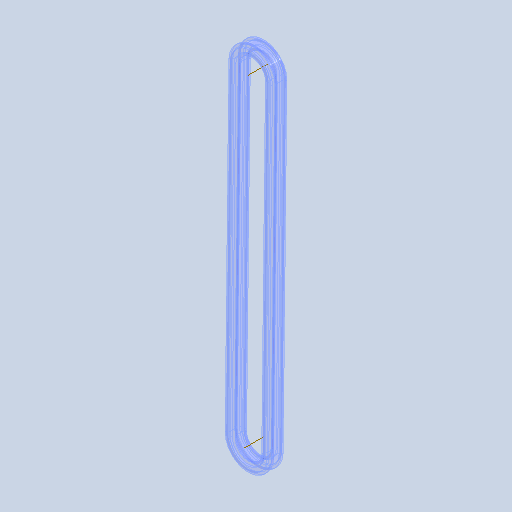
# Autodesk Inventor part: Cadena de rodillos
Saved by Autodesk Inventor 2022.1 (Build 261234000, 234)
## iProperties
Created: 2021-09-11
Part Number: Cadena de rodillos
Material: Generic
Document SubType Name: Modeling
Designer: seb_0
Density: 1 g/cm^3
Appearance: Clear - Blue
CustomPartVersion: 1
Author: seb_0
Autodesk Inventor part; units mm, degrees
ref_plane "Plano de trabajo2" through (36.0243, 99.5749, 0) normal (-1, 0, 0) x (0, 0, 1)
ref_plane "Plano de trabajo3" through (27.084, -687.8643, 0) normal (0.415415, 0.909632, 0) x (0, 0, 1)
sketch "Trayectoria" plane through (0, 0, 0) normal (0, 0, 1) x (1, 0, 0)
  arc A0 (80.3897, 99.0711) -> (-8.3412, 100.0786) centre (36.0243, 99.5749) ccw
  arc A1 (-17.2814, -687.3606) -> (71.4495, -688.3681) centre (27.084, -687.8643) ccw
  line L0 (-17.2814, -687.3606) -> (-8.3412, 100.0786)
  line L1 (80.3897, 99.0711) -> (71.4495, -688.3681)
  dimension "d31" = 24
  constraints: 4 end point, 4 point on circle, 2 centre point
ref_plane "Plano de sección" through (-8.3412, 100.0786, 0) normal (-0.0113528, -0.9999356, 0) x (0, 0, 1)
sketch "Boceto de sección" plane through (-8.3412, 100.0786, 0) normal (-0.0113528, -0.9999356, 0) x (0, 0, 1)
  line L0 (-18, -5) -> (18, -5)
  line L1 (18, -5) -> (18, 5)
  line L2 (18, 5) -> (-18, 5)
  line L3 (-18, 5) -> (-18, -5)
  line L4 (-9, -7.5) -> (9, -7.5)
  line L5 (9, -7.5) -> (9, 7.5)
  line L6 (9, 7.5) -> (-9, 7.5)
  line L7 (-9, 7.5) -> (-9, -7.5)
  line L8 (-9, 0) -> (9, 0) construction
  line L9 (-14, -12) -> (-9, -12)
  line L10 (-9, -12) -> (-9, 12)
  line L11 (-9, 12) -> (-14, 12)
  line L12 (-14, 12) -> (-14, -12)
  line L13 (9, -12) -> (14, -12)
  line L14 (14, -12) -> (14, 12)
  line L15 (14, 12) -> (9, 12)
  line L16 (9, 12) -> (9, -12)
  line L17 (-18, 0) -> (18, 0) construction
  point P0 (0, 0)
  point P1 (0, 0)
  dimension "d21" = 10
  dimension "d22" = 15
  dimension "d23" = 18
  dimension "d24" = 5
  dimension "d31" = 24
  dimension "d32" = 36
  constraints: 36 end point, 8 midpoint, 8 parallel, 4 horizontal, 4 perpendicular, 3 collinear, 1 coincident, 1 other
  measures "d21" distance between parallel lines of L2 L0
  measures "d22" distance between parallel lines of L6 L4
  measures "d23" distance between parallel lines of L5 L7
  measures "d24" distance between parallel lines of L12 L10
  measures "d31" distance between parallel lines of L11 L9
  measures "d32" distance between parallel lines of L1 L3
sweep "Sólido" add profiles "Boceto de sección" path "Trayectoria" path curves L1 A1 L0 A0
pattern_of_one "Strand Pattern"
equation "\"d21\" = da_d2"
equation "\"d22\" = da_d1"
equation "\"d23\" = da_b1"
equation "\"d24\" = da_t1 + da_t2"
equation "\"d30\" = da_pt"
equation "\"da_p\" = 25"
equation "\"da_b1\" = 18"
equation "\"da_h2\" = 24"
equation "\"da_h3\" = 24"
equation "\"da_d1\" = 15"
equation "\"da_d2\" = 10"
equation "\"da_pt\" = 32"
equation "\"da_b\" = 36"
equation "\"da_t1\" = 2.5"
equation "\"da_t2\" = 2.5"
body "Solid1"
